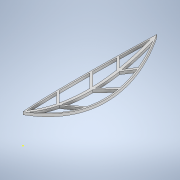
# Autodesk Inventor part: Part2
Saved by Autodesk Inventor 2020.2 (Build 242310000, 310)
## iProperties
Created: 2020-02-19
Part Number: Part2
Material: Generic
Document SubType Name: Modeling
Designer: lenovo
Density: 1 g/cm^3
Appearance: Default
Author: lenovo
Autodesk Inventor part; units mm, degrees
ref_plane "YZ Plane" through (0, 0, 0) normal (1, 0, 0) x (0, 1, 0)
ref_plane "XZ Plane" through (0, 0, 0) normal (0, 1, 0) x (-1, 0, 0)
ref_plane "XY Plane" through (0, 0, 0) normal (0, 0, 1) x (1, 0, 0)
sketch "Sketch1" plane through (0, 0, 0) normal (0, 1, 0) x (-1, 0, 0)
  arc A0 (0, -50) -> (0, 0) centre (-48.9898, -25) ccw
  arc A1 (0, -49) -> (0, -1) centre (-49.4874, -25) ccw
  line L0 (0, 0) -> (0, -50)
  line L1 (0, -12.5) -> (5.5721, -18.0721)
  line L2 (0, -12.5) -> (7.8802, -12.5) construction
  line L3 (0, -13.5) -> (5.704, -19.204)
  line L4 (0, -25) -> (5.7127, -30.7127)
  line L5 (0, -25) -> (8.079, -25) construction
  line L6 (0, -26) -> (5.6114, -31.6114)
  line L7 (0, -35) -> (4.157, -39.157)
  line L8 (0, -35) -> (5.8789, -35) construction
  line L9 (0, -36) -> (3.9417, -39.9417)
  arc A2 (0, 0) -> (0, -50) centre (48.9898, -25) ccw
  arc A3 (0, -1) -> (0, -49) centre (49.4874, -25) ccw
  line L10 (0, -12.5) -> (-5.5721, -18.0721)
  line L11 (0, -13.5) -> (-5.704, -19.204)
  line L12 (0, -25) -> (-5.7127, -30.7127)
  line L13 (0, -26) -> (-5.6114, -31.6114)
  line L14 (0, -35) -> (-4.157, -39.157)
  line L15 (0, -36) -> (-3.9417, -39.9417)
  line L16 (0.5, 0) -> (0.5, -50.0047)
  line L17 (-0.5, 0) -> (-0.5, -50.0047)
  point P0 (5.1659, -31.1659)
  point P1 (3.7628, -38.7628)
  point P2 (0.5, -35.5)
  point P3 (0.5, -26.5)
  point P4 (-3.7628, -38.7628)
  point P5 (-5.1659, -31.1659)
  point P6 (-0.5, -26.5)
  point P7 (-0.5, -35.5)
  point P8 (-5.2605, -30.2605)
  point P9 (-5.1441, -18.6441)
  point P10 (-0.5, -14)
  point P11 (-0.5, -25.5)
  point P12 (-4.9987, -17.4987)
  point P13 (-0.5, -2.0596)
  point P14 (-0.5, -13)
  point P15 (-0.5, -36.5)
  point P16 (-0.5, -47.9404)
  point P17 (-3.5525, -39.5525)
  point P18 (4.9987, -17.4987)
  point P19 (0.5, -13)
  point P20 (0.5, -2.0596)
  point P21 (3.5525, -39.5525)
  point P22 (0.5, -47.9404)
  point P23 (0.5, -36.5)
  point P24 (5.1441, -18.6441)
  point P25 (5.2605, -30.2605)
  point P26 (0.5, -25.5)
  point P27 (0.5, -14)
  dimension "d0" = 50
  dimension "d1" = 55
  dimension "d2" = 48
  dimension "d3" = 55
  dimension "d4" = 45
  dimension "d5" = 45
  dimension "d6" = 45
  constraints: 36 end point, 20 point on circle, 10 symmetric about line, 4 centre point, 4 parallel, 4 point on line, 3 equal length, 3 horizontal, 1 midpoint, 1 vertical, 2 other
  measures "d0" distance of L0.start L0.end
  measures "d1" radius of A0
  measures "d2" distance of A1.end A1.start
  measures "d3" radius of A1
  measures "d4" angle of L1 L2
  measures "d5" angle of L4 L5
  measures "d6" angle of L7 L8
extrude "Extrusion1" add sketch "Sketch1" along normal blind 20 contours L9 A1 L7 A0 | A0 L16 A1 L9 | L7 A1 L6 A0 | A0 L0 A1 L16 | L9 L16 L7 A1 | L6 A1 L4 A0 | A2 L17 A3 L0 | A1 L0 L9 L16 | L9 L0 L7 L16 | L4 A1 L3 A0 | L6 L16 L4 A1 | L7 L0 L6 L16 | A3 L17 L15 L0 | A2 L15 A3 L17 | L15 L17 L14 L0 | L3 A1 L1 A0 | L6 L0 L4 L16 | L14 L17 L13 L0 | A2 L14 A3 L15 | L15 A3 L14 L17 | L1 A1 L16 A0 | L3 L16 L1 A1 | L4 L0 L3 L16 | L13 L17 L12 L0 | A2 L13 A3 L14 | L16 A1 L0 A0 | L3 L0 L1 L16 | L12 L17 L11 L0 | L13 A3 L12 L17 | A2 L12 A3 L13 | L0 A3 L17 A2 | L16 L1 L0 A1 | L11 L17 L10 L0 | A2 L11 A3 L12 | L0 L10 L17 A3 | L17 A3 L10 A2 | L11 A3 L10 L17 | A2 L10 A3 L11
sketch "Sketch2" plane through (0, 0, 0) normal (0, 0, 1) x (1, 0, 0)
  point P0 (0, 0)
sketch "Sketch3" plane through (0, 0, 0) normal (1, 0, 0) x (0, 1, 0)
  line L0 (0, 0) -> (20, 0) projected
  line L1 (0, -50) -> (20, -50) projected
  arc A0 (10, 0) -> (10, -50) centre (64.5436, -25) ccw
  arc A1 (11, 0) -> (11, -50) centre (65.5436, -25) ccw
  line L2 (11, 0) -> (11, -50) construction
  line L3 (11, 0) -> (61, 0) construction
  line L4 (11, 0) -> (20, 0)
  line L5 (20, -50) -> (20, 0) projected
  line L6 (20, 0) -> (20, -50)
  line L7 (20, -50) -> (11, -50)
  line L8 (10, 0) -> (0, 0)
  line L9 (0, 0) -> (0, -50)
  line L10 (10, -50) -> (0, -50)
  point P0 (11, 0)
  point P1 (11, -50)
  dimension "d9" = 60
  dimension "d10" = 50
  dimension "d11" = 90
  dimension "d12" = 60
  constraints: 16 end point, 4 collinear, 4 point on circle, 2 centre point, 2 midpoint, 1 horizontal, 1 perpendicular, 1 vertical
  measures "d9" radius of A0
  measures "d10" distance of L2.start L2.end
  measures "d11" angle of L2 L3
  measures "d12" radius of A1
extrude "Extrusion2" cut sketch "Sketch3" along normal mid plane 20 contours L0 A0 L1 L9 | L0 L5 L1 A1
body "Solid1"
